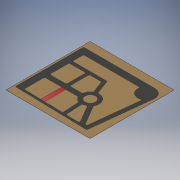
# Autodesk Inventor part: Mcity track
Saved by Autodesk Inventor 2019 (Build 230136000, 136)
## iProperties
Created: 2020-05-05
Part Number: Mcity track
Material: Generic
Document SubType Name: Modeling
Designer: close
Density: 1 g/cm^3
Appearance: Particle Board
Author: close
Autodesk Inventor part; units mm, degrees
ref_plane "YZ Plane" through (0, 0, 0) normal (1, 0, 0) x (0, 1, 0)
ref_plane "XZ Plane" through (0, 0, 0) normal (0, 1, 0) x (-1, 0, 0)
ref_plane "XY Plane" through (0, 0, 0) normal (0, 0, 1) x (1, 0, 0)
sketch "Sketch1" plane through (0, 0, 0) normal (0, 1, 0) x (-1, 0, 0)
  line L0 (0, 0) -> (15240, 0)
  line L1 (15240, 0) -> (15240, -15240)
  line L2 (15240, -15240) -> (0, -15240)
  line L3 (0, -15240) -> (0, 0)
  dimension "d0" = 15240
  dimension "d1" = 15240
  constraints: 8 end point, 2 parallel, 1 horizontal, 1 perpendicular
  measures "d0" distance of L0.start L0.end
  measures "d1" distance of L2.end L0.start
extrude "Extrusion1" add sketch "Sketch1" along normal blind 25.4
sketch "Sketch2" plane through (0, 25.4, 0) normal (0, 1, 0) x (1, 0, 0)
  line L0 (-14935.2, 1562.0729) -> (-14935.2, 13559.8402)
  line L1 (-14736.8176, 1358.93) -> (-1817.9841, 1052.5545)
  line L2 (-1611.2356, 1233.0221) -> (-406.4, 11962.5108)
  line L3 (-2016.0607, 13763.0402) -> (-14732, 13763.0402)
  line L4 (-2315.0035, 1935.1122) -> (-1352.8633, 10503.3117)
  line L5 (-3686.2075, 12543.8402) -> (-13512.8, 12543.8402)
  line L6 (-13716, 12340.6402) -> (-13716, 10747.6666)
  line L7 (-13512.8, 10544.4666) -> (-7552.4546, 10544.4666)
  line L8 (-7361.709, 10411.312) -> (-6460.5488, 7957.2969)
  line L9 (-13512.8, 6403.6024) -> (-10886.8043, 6403.6024)
  line L10 (-10683.6043, 6606.8024) -> (-10683.6043, 9731.6666)
  line L11 (-13512.8, 5489.2024) -> (-10683.6043, 5489.2024)
  line L12 (-10683.6043, 5489.2024) -> (-9414.0453, 5489.2024)
  line L13 (-9414.0453, 5489.2024) -> (-7775.8091, 5489.2024)
  line L14 (-7978.0008, 9934.8666) -> (-9870.8043, 9934.8666)
  line L15 (-10074.0043, 9731.6666) -> (-10074.0043, 6606.8024)
  line L16 (-9870.8043, 6403.6024) -> (-7941.5651, 6403.6024)
  line L17 (-13716, 6606.8024) -> (-13716, 9731.6666)
  line L18 (-13512.8, 9934.8666) -> (-10886.8043, 9934.8666)
  line L19 (-13716, 1966.2624) -> (-13716, 5286.0024)
  line L20 (-5265.9143, 4746.921) -> (-3564.6116, 1837.0583)
  line L21 (-4719.0152, 5321.5764) -> (-2692.3523, 1855.2262)
  line L22 (-7787.2552, 9801.712) -> (-7037.5702, 7760.1901)
  line L23 (-15240, 15240) -> (-15240, 0) projected
  line L24 (-6571.3344, 1817.9516) -> (-6725.3675, 4535.8332)
  line L25 (-5930.4882, 1770.1358) -> (-6084.9684, 4495.908)
  arc A0 (-7600.1322, 5388.1194) -> (-6845.407, 4709.885) centre (-6172.0298, 6218.2437) ccw
  arc A1 (-5916.0462, 4707.7491) -> (-5526.8987, 4828.6656) centre (-6172.0298, 6218.2437) ccw
  arc A2 (-4726.2381, 5513.2025) -> (-6258.8372, 7824.4383) centre (-6172.0298, 6218.2437) ccw
  arc A3 (-7109.8425, 7525.0559) -> (-7743.0935, 6563.2215) centre (-6172.0298, 6218.2437) ccw
  arc A4 (-3484.4118, 12316.7921) -> (-1610.5268, 10721.3945) centre (-2016.0607, 12143.2628) ccw
  arc A5 (-406.4, 11962.5108) -> (-2016.0607, 13763.0402) centre (-2016.0607, 12143.2628) ccw
  arc A6 (-13512.8, 5489.2024) -> (-13716, 5286.0024) centre (-13512.8, 5286.0024) ccw
  arc A7 (-13716, 6606.8024) -> (-13512.8, 6403.6024) centre (-13512.8, 6606.8024) ccw
  arc A8 (-10886.8043, 6403.6024) -> (-10683.6043, 6606.8024) centre (-10886.8043, 6606.8024) ccw
  arc A9 (-10074.0043, 6606.8024) -> (-9870.8043, 6403.6024) centre (-9870.8043, 6606.8024) ccw
  arc A10 (-10683.6043, 9731.6666) -> (-10886.8043, 9934.8666) centre (-10886.8043, 9731.6666) ccw
  arc A11 (-9870.8043, 9934.8666) -> (-10074.0043, 9731.6666) centre (-9870.8043, 9731.6666) ccw
  arc A12 (-7787.2552, 9801.712) -> (-7978.0008, 9934.8666) centre (-7978.0008, 9731.6666) ccw
  arc A13 (-7361.709, 10411.312) -> (-7552.4546, 10544.4666) centre (-7552.4546, 10341.2666) ccw
  arc A14 (-13512.8, 9934.8666) -> (-13716, 9731.6666) centre (-13512.8, 9731.6666) ccw
  arc A15 (-13716, 10747.6666) -> (-13512.8, 10544.4666) centre (-13512.8, 10747.6666) ccw
  arc A16 (-13716, 1966.2624) -> (-13517.6176, 1763.1195) centre (-13512.8, 1966.2624) ccw
  arc A17 (-7600.1322, 5388.1194) -> (-7775.8091, 5489.2024) centre (-7775.8091, 5286.0024) ccw
  arc A18 (-7941.5651, 6403.6024) -> (-7743.0935, 6563.2215) centre (-7941.5651, 6606.8024) ccw
  arc A19 (-7109.8425, 7525.0559) -> (-7037.5702, 7760.1901) centre (-7228.3158, 7690.1447) ccw
  arc A20 (-6460.5488, 7957.2969) -> (-6258.8372, 7824.4383) centre (-6269.8032, 8027.3422) ccw
  arc A21 (-3484.4118, 12316.7921) -> (-3686.2075, 12543.8402) centre (-3686.2075, 12340.6402) ccw
  arc A22 (-1352.8633, 10503.3117) -> (-1610.5268, 10721.3945) centre (-1554.7942, 10525.9869) ccw
  arc A23 (-13512.8, 12543.8402) -> (-13716, 12340.6402) centre (-13512.8, 12340.6402) ccw
  arc A24 (-14732, 13763.0402) -> (-14935.2, 13559.8402) centre (-14732, 13559.8402) ccw
  arc A25 (-14935.2, 1562.0729) -> (-14736.8176, 1358.93) centre (-14732, 1562.0729) ccw
  arc A26 (-1817.9841, 1052.5545) -> (-1611.2356, 1233.0221) centre (-1813.1665, 1255.6974) ccw
  line L26 (-13517.6176, 1763.1195) -> (-6779.0265, 1603.311)
  line L27 (-5732.4314, 1578.4906) -> (-3744.8471, 1531.3542)
  arc A27 (-6779.0265, 1603.311) -> (-6571.3344, 1817.9516) centre (-6774.2089, 1806.4539) ccw
  arc A28 (-5930.4882, 1770.1358) -> (-5732.4314, 1578.4906) centre (-5727.6138, 1781.6335) ccw
  arc A29 (-3744.8471, 1531.3542) -> (-3564.6116, 1837.0583) centre (-3740.0295, 1734.4971) ccw
  arc A30 (-2692.3523, 1855.2262) -> (-2315.0035, 1935.1122) centre (-2516.9343, 1957.7874) ccw
  arc A31 (-4726.2381, 5513.2025) -> (-4719.0152, 5321.5764) centre (-4543.5973, 5424.1376) ccw
  arc A32 (-5265.9143, 4746.921) -> (-5526.8987, 4828.6656) centre (-5441.3322, 4644.3598) ccw
  arc A33 (-5916.0462, 4707.7491) -> (-6084.9684, 4495.908) centre (-5882.094, 4507.4057) ccw
  arc A34 (-6725.3675, 4535.8332) -> (-6845.407, 4709.885) centre (-6928.2419, 4524.3355) ccw
  line L28 (0, 0) -> (0, 15240) projected
  point P0 (-3439.3334, 12543.8402)
  point P1 (-6406.322, 7809.628)
  point P2 (-7654.2854, 5489.2024)
  point P3 (-7769.8073, 6403.6024)
  point P4 (-5364.833, 4916.109)
  point P5 (-4776.041, 5419.1118)
  point P6 (-6981.7147, 7608.0859)
  point P7 (-6732.6566, 4664.4482)
  point P8 (-6095.8611, 4688.1065)
  point P9 (-1314.8846, 10841.5257)
  dimension "d4" = 304.8
  dimension "d5" = 1219.2
  dimension "d6" = 1219.2
  dimension "d7" = 1219.2
  dimension "d8" = 1219.2
  dimension "d9" = 609.6
  dimension "d10" = 914.4
  dimension "d11" = 609.6
  dimension "d12" = 914.4
  dimension "d14" = 609.6
  dimension "d16" = 203.2
  dimension "d17" = 609.6
  dimension "d18" = 203.2
  dimension "d19" = 203.2
  dimension "d20" = 406.4
  constraints: 80 point on circle, 61 tangent, 54 end point, 35 centre point, 26 equal radius, 13 point on line, 6 parallel, 5 horizontal, 5 perpendicular, 3 vertical
  measures "d4" distance between parallel lines of L23 L0
  measures "d5" distance between parallel lines of L19 L0
  measures "d6" distance between parallel lines of L0 L17
  measures "d7" distance between parallel lines of L0 L6
  measures "d8" distance between parallel lines of L3 L5
  measures "d9" distance between parallel lines of L7 L18
  measures "d10" distance between parallel lines of L9 L11
  measures "d11" distance between parallel lines of L15 L10
  measures "d12" distance between parallel lines of L16 L13
  measures "d14" distance between parallel lines of L8 L22
  measures "d16" radius of A6
  measures "d17" distance between parallel lines of L7 L14
  measures "d18" radius of A11
  measures "d19" radius of A27
  measures "d20" distance from line of L28 L2.end
extrude "Extrusion2" add sketch "Sketch2" along normal blind 0.254
sketch "Sketch3" plane through (0, 25.4, 0) normal (0, 1, 0) x (1, 0, 0)
  line L0 (-13512.8, 5489.2024) -> (-7775.8091, 5489.2024) projected
  line L1 (-10644.3045, 5489.2024) -> (-10644.3045, 1694.9777)
  line L2 (-6779.0265, 1603.311) -> (-13517.6176, 1763.1195) projected
  line L3 (-9869.7738, 1676.6094) -> (-9869.7738, 5489.2024)
  line L4 (-10644.3045, 5489.2024) -> (-9869.7738, 5489.2024)
  line L5 (-9869.7738, 1676.6094) -> (-10644.3045, 1694.9777)
  point P0 (0, 0)
  constraints: 8 end point, 2 collinear, 2 vertical, 1 midpoint, 1 point on line
extrude "Extrusion3" cut sketch "Sketch3" against normal blind 1.27
sketch "Sketch4" plane through (0, 25.654, 0) normal (0, 1, 0) x (1, 0, 0)
  arc A0 (-4726.2381, 5513.2025) -> (-6258.8372, 7824.4383) centre (-6172.0298, 6218.2437) ccw projected
  circle A1 centre (-6172.0298, 6218.2437) radius 933.3587
  point P0 (0, 0)
  constraints: 1 centre point, 1 coincident
extrude "Extrusion4" add sketch "Sketch4" along normal blind 1.27
equation "\"d6\" = d5"
equation "\"d7\" = d6"
equation "\"d8\" = d7"
equation "\"d12\" = d10"
equation "\"d14\" = d9"
equation "\"d17\" = d14"
body "Solid1"
